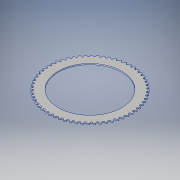
# Autodesk Inventor part: Turret Gear
Saved by Autodesk Inventor 2019.4 (Build 234330000, 330)
## iProperties
Created: 2020-01-22
Part Number: Turret Gear
Material: Aluminum 6061
Document SubType Name: Modeling
Designer: admin
Density: 2.7 g/cm^3
Appearance: Aluminum - Flat
Author: admin
Autodesk Inventor part; units mm, degrees
ref_plane "YZ Plane" through (0, 0, 0) normal (1, 0, 0) x (0, 1, 0)
ref_plane "XZ Plane" through (0, 0, 0) normal (0, 1, 0) x (-1, 0, 0)
ref_plane "XY Plane" through (0, 0, 0) normal (0, 0, 1) x (1, 0, 0)
sketch "Sketch1" plane through (0, 0, 0) normal (0, 1, 0) x (-1, 0, 0)
  circle A0 centre (0, 0) radius 175 construction
  circle A1 centre (0, 0) radius 191.0078 construction
  arc A2 (186.7668, -40.0266) -> (184.3529, -49.7289) centre (185.6551, -44.9015) ccw
  arc A3 (181.4977, -59.309) -> (184.3529, -49.7289) centre (183.0507, -54.5564) ccw
  arc A4 (181.4977, -59.309) -> (178.1449, -68.7266) centre (179.9446, -64.0617) ccw
  arc A5 (174.3039, -77.9558) -> (178.1449, -68.7266) centre (176.3453, -73.3915) ccw
  arc A6 (174.3039, -77.9558) -> (168.0369, -85.1929) centre (172.2626, -82.5201) ccw
  line L0 (0, 0) -> (187.8424, -55.9845)
  line L1 (0, 0) -> (180.9614, -75.3127)
  dimension "d0" = 350
  dimension "d1" = 5
  dimension "d2" = 5
  dimension "d3" = 5
  dimension "d4" = 5
  dimension "d5" = 5
  dimension "d6" = 6
  constraints: 18 point on circle, 7 centre point, 4 end point, 4 equal radius, 2 coincident
  measures "d0" diameter of A0
  measures "d1" radius of A2
  measures "d2" radius of A3
  measures "d3" radius of A4
  measures "d4" radius of A5
  measures "d5" radius of A6
  measures "d6" angle of L0 L1
extrude "Extrusion1" add sketch "Sketch1" along normal blind 5
pattern_circular "Circular Pattern1" count 60 over 360 about axis through (0, 0, 0) along (0, 1, 0) of "Extrusion1"
sketch "Sketch2" plane through (0, 5, 0) normal (0, 1, 0) x (1, 0, 0)
  circle A0 centre (0, 0) radius 148
  dimension "d12" = 296
  constraints: 1 centre point, 1 coincident
  measures "d12" diameter of A0
extrude "Extrusion2" cut sketch "Sketch2" against normal through all
body "Solid1"
